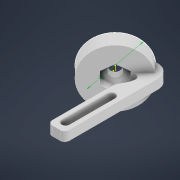
# Autodesk Inventor part: arm
Saved by Autodesk Inventor 2021.2 (Build 252289000, 289)
## iProperties
Created: 2021-01-20
Part Number: arm
Material: Generic
Document SubType Name: Modeling
Designer: Administrator
Density: 1 g/cm^3
Appearance: Default
Author: Administrator
Autodesk Inventor part; units mm, degrees
note: some values were not read from the file. Chosen so that the rebuilt part matches the saved one: direction of "Hole1".
ref_plane "YZ Plane" through (0, 0, 0) normal (1, 0, 0) x (0, 1, 0)
ref_plane "XZ Plane" through (0, 0, 0) normal (0, 1, 0) x (-1, 0, 0)
ref_plane "XY Plane" through (0, 0, 0) normal (0, 0, 1) x (1, 0, 0)
sketch "Sketch1" plane through (0, 0, 0) normal (0, 1, 0) x (-1, 0, 0)
  line L0 (-3.75, -25) -> (-3.75, 23)
  line L1 (-1.75, 25) -> (1.75, 25)
  line L2 (3.75, 23) -> (3.75, -25)
  line L3 (3.75, -25) -> (-3.75, -25)
  line L4 (-3.75, -25) -> (3.75, 25) construction
  line L5 (-3.75, 25) -> (3.75, -25) construction
  line L6 (0, 0.8712) -> (0, 20.8712) construction
  line L7 (-1.7, 0.8712) -> (-1.7, 20.8712)
  line L8 (1.7, 20.8712) -> (1.7, 0.8712)
  arc A0 (-1.7, 0.8712) -> (1.7, 0.8712) centre (0, 0.8712) ccw
  arc A1 (1.7, 20.8712) -> (-1.7, 20.8712) centre (0, 20.8712) ccw
  arc A2 (3.75, 23) -> (1.75, 25) centre (1.75, 23) ccw
  arc A3 (-1.75, 25) -> (-3.75, 23) centre (-1.75, 23) ccw
  line L9 (-3.75, -25) -> (12.9085, -8.3415)
  line L10 (12.9085, -8.3415) -> (15.4834, -10.9164)
  line L11 (15.4834, -10.9164) -> (-1.1751, -27.5749)
  line L12 (-1.1751, -27.5749) -> (-3.75, -25)
  arc A4 (3.75, -4.8061) -> (3.75, -20.0848) centre (12.1805, -12.4455) ccw
  point P0 (0, 0)
  point P1 (0, 10.8712)
  point P2 (1.3998, -25)
  point P3 (3.75, -17.5)
  point P4 (2.627, -18.623)
  dimension "d0" = 7.5
  dimension "d1" = 50
  dimension "d2" = 20
  dimension "d3" = 1.7
  dimension "d4" = 2
  dimension "d8" = 45
  constraints: 28 end point, 10 point on circle, 8 tangent, 6 point on line, 5 centre point, 3 midpoint, 3 parallel, 3 perpendicular, 2 vertical, 1 equal radius
  measures "d0" distance between parallel lines of L2 L0
  measures "d1" distance of L4.end L2.end
  measures "d2" distance of L8.start L8.end
  measures "d3" radius of A1
  measures "d4" radius of A2
  measures "d8" angle of L0 L9
extrude "Main Arm" add sketch "Sketch1" along normal blind 4 contours L9 A4 L2 L11 L3 | L0 A3 L1 A2 L2 A4 L9 | L9 L2 A4 | L2 L9 L10 L11 picked at (3.6165, -19.0676)
sketch "Pad holder" plane through (-15.4834, 0, -10.9164) normal (-0.7071068, 0, -0.7071068) x (-0.7071068, 0, 0.7071068)
  line L0 (-3.8154, 0) -> (-3.8154, 4) projected
  circle A0 centre (-3.8154, 2) radius 12.5
  point P0 (-3.2294, 0)
  dimension "d9" = 25
  constraints: 1 centre point, 1 coincident, 1 midpoint
  measures "d9" diameter of A0
extrude "pad area" add sketch "Pad holder" against normal blind 7
hole "Hole1" at (-12.7855, 2, -13.6143) direction (0.7071068, 0, 0.7071068) diameter 5.0038 depth 7
sketch "Screw position" plane through (-10.5337, 0, -5.9666) normal (0.7071068, 0, 0.7071068) x (0.7071068, 0, -0.7071068)
  line L0 (3.8154, 0) -> (3.8154, 4) projected
  line L1 (3.8154, 7.4848) -> (8.5654, 4.7424)
  line L2 (8.5654, 4.7424) -> (8.5654, -0.7424)
  line L3 (8.5654, -0.7424) -> (3.8154, -3.4848)
  line L4 (3.8154, -3.4848) -> (-0.9346, -0.7424)
  line L5 (-0.9346, -0.7424) -> (-0.9346, 4.7424)
  line L6 (-0.9346, 4.7424) -> (3.8154, 7.4848)
  point P0 (3.2294, 0)
  point P1 (3.8154, 2)
  dimension "d21" = 9.5
  constraints: 12 end point, 1 midpoint, 1 vertical, 13 other
  measures "d21" distance between parallel lines of L2 L5
extrude "Extrusion3" cut sketch "Screw position" against normal blind 4
fillet "Fillet1" radius 6 3 edges at (-1.3998, 2, -25) (3.75, 2, -25) (-3.75, 2, -4.8061)
fillet "Fillet2" radius 2 1 edges at (-1.1744, 2, -15.326)
body "Solid1"
